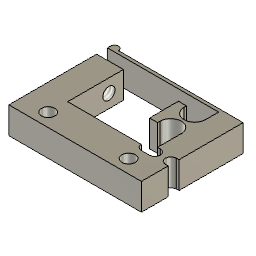
piezo_actuator_mount (Autodesk Fusion 360 design; units mm, degrees)
part number: 2025-08-01-23-50-47-375
Autodesk Fusion 360 part; units mm, degrees
note: some values were not read from the file. Chosen so that the rebuilt part matches the saved one: how an offset face is resized.
sketch "Sketch1" plane through (0, 0, 0) normal (0, 0, 1) x (1, 0, 0)
  line L0 (-12.375, 9.5) -> (12.375, 9.5)
  line L1 (12.375, 9.5) -> (12.375, -9.5)
  line L2 (12.375, -9.5) -> (-12.375, -9.5)
  line L3 (-12.375, -9.5) -> (-12.375, 9.5)
  line L4 (-12.375, 9.5) -> (12.375, -9.5) construction
  line L5 (12.375, 9.5) -> (-12.375, -9.5) construction
  line L6 (-7.375, 6.9) -> (2.875, 6.9)
  line L7 (2.875, 6.9) -> (2.875, -3.5)
  line L8 (2.875, -3.5) -> (-7.375, -3.5)
  line L9 (-7.375, -3.5) -> (-7.375, 6.9)
  line L10 (-12.375, 8.9) -> (8.375, 8.9)
  line L11 (8.375, 8.9) -> (8.375, 6.9)
  line L12 (8.375, 6.9) -> (-12.375, 6.9)
  line L13 (-12.375, 6.9) -> (-12.375, 8.9)
  arc A0 (-10.875, 9.5) -> (-12.375, 9.5) centre (-11.625, 9.5) ccw
  line L14 (2.875, 1.5) -> (8.375, 1.5)
  line L15 (8.375, 1.5) -> (8.375, -3.5)
  line L16 (8.375, -3.5) -> (2.875, -3.5)
  line L17 (2.875, -3.5) -> (2.875, 1.5)
  line L18 (7.375, -4.5) -> (8.875, -4.5)
  arc A1 (8.875, -4.5) -> (8.875, -2.5) centre (8.875, -3.5) ccw
  line L19 (8.875, -2.5) -> (7.375, -2.5)
  arc A2 (7.375, -2.5) -> (7.375, -4.5) centre (7.375, -3.5) ccw
  line L20 (11.875, -4.5) -> (13.375, -4.5)
  arc A3 (13.375, -4.5) -> (13.375, -2.5) centre (13.375, -3.5) ccw
  line L21 (13.375, -2.5) -> (11.875, -2.5)
  arc A4 (11.875, -2.5) -> (11.875, -4.5) centre (11.875, -3.5) ccw
  line L22 (11.875, -3.5) -> (13.375, -3.5) construction
  line L23 (4.375, 8.45) -> (4.375, 6.45)
  arc A5 (4.375, 6.45) -> (8.375, 6.45) centre (6.375, 6.45) ccw
  line L24 (8.375, 6.45) -> (8.375, 8.45)
  arc A6 (8.375, 8.45) -> (4.375, 8.45) centre (6.375, 8.45) ccw
  line L25 (6.375, 8.45) -> (6.375, 6.45) construction
  line L26 (4.375, 1.95) -> (4.375, -0.05)
  arc A7 (4.375, -0.05) -> (8.375, -0.05) centre (6.375, -0.05) ccw
  line L27 (8.375, -0.05) -> (8.375, 1.95)
  arc A8 (8.375, 1.95) -> (4.375, 1.95) centre (6.375, 1.95) ccw
  line L28 (6.375, 1.95) -> (6.375, -0.05) construction
  circle A9 centre (-7.5, -7) radius 1.25
  circle A10 centre (7.5, -7) radius 1.25
  dimension "d2" = 19
  dimension "d3" = 2
  dimension "d4" = 10.25
  dimension "d5" = 6
  dimension "d7" = 10.4
  dimension "d8" = 20.75
  dimension "d9" = 0.75
  dimension "d10" = 5.5
  dimension "d11" = 5
  dimension "d12" = 1
  dimension "d13" = 3
  dimension "d15" = 6
  dimension "d16" = 1.5
  dimension "d17" = 2
  dimension "d18" = 2
  dimension "d19" = 1.5
  dimension "d20" = 4.5
  dimension "d21" = 5.4
  dimension "d22" = 0.45
  dimension "d27" = 4
  dimension "d28" = 0.5
  dimension "d29" = 2.5
  dimension "d30" = 2.5
  dimension "d31" = 15
  dimension "d32" = 24.75
  dimension "d33" = 4.875
  constraint horizontal L0
  constraint perpendicular L0 L1
  constraint parallel L0 L2
  constraint parallel L1 L3
  constraint coincident L4 origin
  constraint coincident L5 origin
  constraint horizontal L6
  constraint vertical L7
  constraint horizontal L8
  constraint vertical L9
  constraint horizontal L10
  constraint vertical L11
  constraint horizontal L12
  constraint vertical L13
  constraint collinear L6 L12
  constraint collinear L3 L13
  constraint tangent L3 A0
  constraint coincident L0 A0.start
  constraint horizontal L14
  constraint vertical L15
  constraint horizontal L16
  constraint vertical L17
  constraint collinear L8 L16
  constraint collinear L7 L17
  constraint tangent L18 A1
  constraint tangent A1 L19
  constraint parallel L18 L19
  constraint tangent L19 A2
  constraint tangent L18 A2
  constraint tangent L20 A3
  constraint tangent A3 L21
  constraint parallel L20 L21
  constraint tangent L21 A4
  constraint tangent L20 A4
  constraint perpendicular L1 L22
  constraint equal A1 A4
  constraint horizontal A1.centre A4.centre
  constraint equal L19 L21
  constraint tangent L23 A5
  constraint tangent A5 L24
  constraint parallel L23 L24
  constraint tangent L24 A6
  constraint tangent L23 A6
  constraint perpendicular L12 L25
  constraint tangent L26 A7
  constraint tangent A7 L27
  constraint parallel L26 L27
  constraint tangent L27 A8
  constraint tangent L26 A8
  constraint perpendicular L14 L28
  constraint vertical A5.centre A8.centre
  constraint equal L24 L27
  constraint equal A6 A8
  constraint horizontal A2.centre A4.centre
  constraint collinear L11 L15
  constraint equal A9 A10
  constraint horizontal A9.centre A10.centre
  measures "d2" distance of L0.start L2.end
  measures "d3" distance of L10.end L11.end
  measures "d4" distance of L7.end L8.end
  measures "d5" distance of L2 L8
  measures "d7" distance of L6.start L8.end
  measures "d8" distance of L10.start L10.end
  measures "d9" radius of A0
  measures "d10" distance of L14.start L14.end
  measures "d11" distance of L14.start L7.end
  measures "d12" radius of A4
  measures "d13" distance of A1.centre A4.centre
  measures "d15" distance of L2 A1.centre
  measures "d16" distance of L18.start L18.end
  measures "d17" radius of A6
  measures "d18" distance of A5.end L24.end
  measures "d19" distance of L6.end L23
  measures "d20" distance of A5.centre A8.centre
  measures "d21" distance of L12 L14
  measures "d22" distance of L12 A5.centre
  measures "d27" distance of L1 L15
  measures "d28" distance of L15 A1.centre
  measures "d29" diameter of A10
  measures "d30" distance of L2 A9.centre
  measures "d31" distance of A9.centre A10.centre
  measures "d32" distance of L0.start L0.end
  measures "d33" distance of L3 A9.centre
extrude "Extrude1" add sketch "Sketch1" along normal blind 5 contours L0 A0 | L0 L3 L10 A6 | L0 L10 A6 | L0 L1 L2 L3 L7 L8 L9 L10 L11 L12 L14 L15 L16 L18 A1 L19 A2 L20 L21 A4 L23 A5 L24 A6 L26 L27 A8
sketch "Sketch2" plane through (-12.375, 0, 0) normal (-1, 0, 0) x (0, -1, 0)
  line L0 (-6.9, 0) -> (9.5, 0)
  line L1 (9.5, 0) -> (9.5, 5)
  line L2 (9.5, 5) -> (-6.9, 5)
  line L3 (-6.9, 5) -> (-6.9, 0)
  circle A0 centre (-4.2, 2.5) radius 1.5
  dimension "d34" = 3
  dimension "d35" = 2.7
  dimension "d38" = 5
  dimension "d39" = 2.5
  measures "d34" diameter of A0
  measures "d35" distance of L3 A0.centre
  measures "d38" distance of L0.end L1.end
  measures "d39" distance of L2 A0.centre
extrude "Extrude2" cut sketch "Sketch2" against normal blind 15 contours A0
thread "Thread1" [suppressed]
thread "Thread2" [suppressed]
sketch "Sketch3" plane through (0, 0, 6.35) normal (0, 0, 1) x (-1, 0, 0)
  circle A0 centre (7.5, 7) radius 1.5
  circle A1 centre (-7.5, 7) radius 1.5
  line L0 (-8.375, -1.95) -> (-8.375, 2.5)
  line L1 (-8.375, 2.5) -> (-8.875, 2.5)
  arc A2 (-8.875, 4.5) -> (-8.875, 2.5) centre (-8.875, 3.5) ccw
  line L2 (-8.875, 4.5) -> (-7.375, 4.5)
  arc A3 (-6.375, 3.5) -> (-7.375, 4.5) centre (-7.375, 3.5) ccw
  line L3 (-6.375, 3.5) -> (7.125, 3.5)
  line L4 (7.125, 3.5) -> (7.125, -6.9)
  line L5 (7.125, -6.9) -> (12.375, -6.9)
  line L6 (12.375, -6.9) -> (12.375, 9.5)
  line L7 (12.375, 9.5) -> (-12.375, 9.5)
  line L8 (-12.375, 9.5) -> (-12.375, 4.5)
  line L9 (-12.375, 4.5) -> (-11.875, 4.5)
  arc A4 (-11.875, 2.5) -> (-11.875, 4.5) centre (-11.875, 3.5) ccw
  line L10 (-11.875, 2.5) -> (-12.375, 2.5)
  line L11 (-12.375, 2.5) -> (-12.375, -9.5)
  line L12 (-12.375, -9.5) -> (10.875, -9.5)
  arc A5 (10.875, -9.5) -> (12.375, -9.5) centre (11.625, -9.5) ccw
  line L13 (12.375, -9.5) -> (12.375, -8.9)
  line L14 (12.375, -8.9) -> (-8.375, -8.9)
  line L15 (-8.375, -8.9) -> (-8.375, -6.45)
  arc A6 (-4.375, -6.45) -> (-8.375, -6.45) centre (-6.375, -6.45) ccw
  line L16 (-4.375, -6.45) -> (-4.375, -6.9)
  line L17 (-4.375, -6.9) -> (-2.875, -6.9)
  line L18 (-2.875, -6.9) -> (-2.875, -1.5)
  line L19 (-2.875, -1.5) -> (-4.375, -1.5)
  line L20 (-4.375, -1.5) -> (-4.375, -1.95)
  arc A7 (-8.375, -1.95) -> (-4.375, -1.95) centre (-6.375, -1.95) ccw
  line L21 (12.375, -6.9) -> (9.375, -6.9)
  line L22 (9.375, -6.9) -> (9.375, 9.5)
  line L23 (9.375, 9.5) -> (12.375, 9.5)
  line L24 (12.375, 9.5) -> (12.375, -6.9)
  dimension "d46" = 3
  constraint horizontal L21
  constraint vertical L22
  constraint horizontal L23
  constraint vertical L24
  constraint coincident L7 L22.end
  constraint coincident L5.end L6.start
  measures "d46" distance of L22.end L6.end
extrude "Extrude3" [suppressed]
sketch "Sketch4" plane through (0, 0, 6.35) normal (0, 0, 1) x (-1, 0, 0)
  line L0 (9.375, -6.9) -> (9.375, 9.5)
  line L1 (9.375, 9.5) -> (-12.375, 9.5)
  line L2 (-12.375, 9.5) -> (-12.375, 4.5)
  line L3 (-12.375, 4.5) -> (-11.875, 4.5)
  arc A0 (-11.875, 2.5) -> (-11.875, 4.5) centre (-11.875, 3.5) ccw
  line L4 (-11.875, 2.5) -> (-12.375, 2.5)
  line L5 (-12.375, 2.5) -> (-12.375, -9.5)
  line L6 (-12.375, -9.5) -> (10.875, -9.5)
  arc A1 (10.875, -9.5) -> (12.375, -9.5) centre (11.625, -9.5) ccw
  line L7 (12.375, -9.5) -> (12.375, -8.9)
  line L8 (12.375, -8.9) -> (-8.375, -8.9)
  line L9 (-8.375, -8.9) -> (-8.375, -6.45)
  arc A2 (-4.375, -6.45) -> (-8.375, -6.45) centre (-6.375, -6.45) ccw
  line L10 (-4.375, -6.45) -> (-4.375, -6.9)
  line L11 (-4.375, -6.9) -> (-2.875, -6.9)
  line L12 (-2.875, -6.9) -> (-2.875, -1.5)
  line L13 (-2.875, -1.5) -> (-4.375, -1.5)
  line L14 (-4.375, -1.5) -> (-4.375, -1.95)
  arc A3 (-8.375, -1.95) -> (-4.375, -1.95) centre (-6.375, -1.95) ccw
  line L15 (-8.375, -1.95) -> (-8.375, 2.5)
  line L16 (-8.375, 2.5) -> (-8.875, 2.5)
  arc A4 (-8.875, 4.5) -> (-8.875, 2.5) centre (-8.875, 3.5) ccw
  line L17 (-8.875, 4.5) -> (-7.375, 4.5)
  arc A5 (-6.375, 3.5) -> (-7.375, 4.5) centre (-7.375, 3.5) ccw
  line L18 (-6.375, 3.5) -> (7.125, 3.5)
  line L19 (7.125, 3.5) -> (7.125, -6.9)
  line L20 (7.125, -6.9) -> (9.375, -6.9)
  circle A6 centre (7.5, 7) radius 1.5
  circle A7 centre (-7.5, 7) radius 1.5
  circle A8 centre (7.5, 7) radius 1.25
  constraint concentric A6 A8
thread "Thread3" "ANSI Unified Screw Threads 0.112(#4) 4-40 UNC 4-40 UNC 3B" major diameter 2.8448 minor diameter 2.2708 pitch 0.635 angle 60 resizes the face on face at (-10.7083, 2.7075, 2.3506)
fillet "Fillet2" [suppressed]
equation "d15 = d5"
equation "d22 = ( d21 - d20 ) / 2"
equation "d28 = ( d27 - d13 ) / 2"
equation "d30 = d5 / 2 - 0.5 mm"
equation "d33 = ( d32 - d31 ) / 2"
equation "d35 = ( 5.4 / 2 ) * 1 mm"
equation "d39 = d38 / 2"
